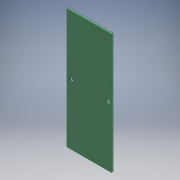
# Autodesk Inventor part: PCB_2
Saved by Autodesk Inventor 2017 (Build 210142000, 142)
## iProperties
Created: 2016-11-21
Part Number: PCB_2
Material: Generic
Document SubType Name: Modeling
Designer: Shichi
Density: 1 g/cm^3
Appearance: Smooth - Dark Sea Green
Author: Shichi
Autodesk Inventor part; units mm, degrees
ref_plane "YZ Plane" through (0, 0, 0) normal (1, 0, 0) x (0, 1, 0)
ref_plane "XZ Plane" through (0, 0, 0) normal (0, 1, 0) x (-1, 0, 0)
ref_plane "XY Plane" through (0, 0, 0) normal (0, 0, 1) x (1, 0, 0)
sketch "Sketch1" plane through (0, 0, 0) normal (0, 1, 0) x (-1, 0, 0)
  line L0 (-13, -35) -> (13, -35)
  line L1 (13, -35) -> (13, 35)
  line L2 (13, 35) -> (-13, 35)
  line L3 (-13, 35) -> (-13, -35)
  line L4 (-13, -35) -> (13, 35) construction
  line L5 (13, -35) -> (-13, 35) construction
  circle A0 centre (10.6, 0) radius 1.25
  circle A1 centre (-11, 0) radius 1.25
  point P0 (0, 0)
  point P1 (13, 0)
  dimension "d0" = 70
  dimension "d1" = 26
  dimension "d2" = 2.5
  dimension "d3" = 21.6
  dimension "d5" = 2.5
  dimension "d8" = 2
  constraints: 12 end point, 3 midpoint, 2 centre point, 2 horizontal alignment, 2 parallel, 1 horizontal, 1 perpendicular
  measures "d0" distance of L0.end L1.end
  measures "d1" distance of L1.end L2.end
  measures "d2" diameter of A0
  measures "d3" distance of A1.centre A0.centre
  measures "d5" diameter of A1
  measures "d8" distance from line of L3 A1.centre
extrude "Extrusion1" add sketch "Sketch1" along normal blind 1
body "Solid1"
